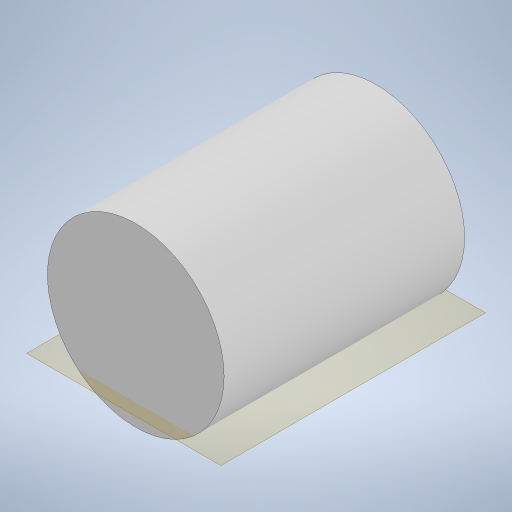
# Autodesk Inventor part: tutorial
Saved by Autodesk Inventor 2023 (Build 270158000, 158)
## iProperties
Created: 2023-03-30
Part Number: tutorial
Material: Ogólny
Document SubType Name: Modeling
Designer: Wiktor
Density: 1 g/cm^3
Appearance: Domyślna
Author: Wiktor
Autodesk Inventor part; units mm, degrees
ref_plane "YZ Plane" through (0, 0, 0) normal (1, 0, 0) x (0, 1, 0)
ref_plane "XY Plane" through (0, 0, 0) normal (0, 0, 1) x (1, 0, 0)
sketch "Szkic1" plane through (0, 0, 0) normal (0, 0, 1) x (1, 0, 0)
  circle A0 centre (0, 0) radius 90
  dimension "d0" = 180
  constraints: 1 centre point, 1 coincident
  measures "d0" diameter of A0
extrude "Wyciągnięcie proste1" add sketch "Szkic1" along normal mid plane 245
ref_plane "Płaszczyzna konstrukcyjna1" through (0, -68, 0) normal (0, 1, 0) x (-1, 0, 0)
